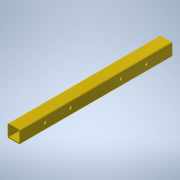
# Autodesk Inventor part: Lacznik prosty
Saved by Autodesk Inventor 2021 (Build 250183000, 183)
## iProperties
Created: 2024-04-08
Part Number: Lacznik prosty
Material: Steel
Document SubType Name: Modeling
Designer: Michal
Density: 7.85 g/cm^3
Appearance: Glossy - Gold
Author: Michal
Autodesk Inventor part; units mm, degrees
ref_plane "YZ Plane" through (0, 0, 0) normal (1, 0, 0) x (0, 1, 0)
ref_plane "XZ Plane" through (0, 0, 0) normal (0, 1, 0) x (-1, 0, 0)
ref_plane "XY Plane" through (0, 0, 0) normal (0, 0, 1) x (1, 0, 0)
sketch "Sketch1" plane through (0, 0, 0) normal (0, 1, 0) x (-1, 0, 0)
  line L0 (-9.5, 11.5) -> (9.5, 11.5) construction
  line L1 (11.5, 9.5) -> (11.5, -9.5) construction
  line L2 (9.5, -11.5) -> (-9.5, -11.5) construction
  line L3 (-11.5, -9.5) -> (-11.5, 9.5) construction
  line L4 (-11.5, 11.5) -> (11.5, -11.5) construction
  line L5 (11.5, 11.5) -> (-11.5, -11.5) construction
  arc A0 (11.5, 9.5) -> (9.5, 11.5) centre (9.5, 9.5) ccw construction
  arc A1 (9.5, -11.5) -> (11.5, -9.5) centre (9.5, -9.5) ccw construction
  arc A2 (-11.5, -9.5) -> (-9.5, -11.5) centre (-9.5, -9.5) ccw construction
  arc A3 (-9.5, 11.5) -> (-11.5, 9.5) centre (-9.5, 9.5) ccw construction
  line L6 (-9.5, -12.5) -> (9.5, -12.5)
  arc A4 (9.5, -12.5) -> (12.5, -9.5) centre (9.5, -9.5) ccw
  line L7 (12.5, -9.5) -> (12.5, 9.5)
  arc A5 (12.5, 9.5) -> (9.5, 12.5) centre (9.5, 9.5) ccw
  line L8 (9.5, 12.5) -> (-9.5, 12.5)
  arc A6 (-9.5, 12.5) -> (-12.5, 9.5) centre (-9.5, 9.5) ccw
  line L9 (-12.5, 9.5) -> (-12.5, -9.5)
  arc A7 (-12.5, -9.5) -> (-9.5, -12.5) centre (-9.5, -9.5) ccw
  line L10 (10.5, -9.5) -> (10.5, 9.5)
  arc A8 (10.5, 9.5) -> (9.5, 10.5) centre (9.5, 9.5) ccw
  line L11 (9.5, 10.5) -> (-9.5, 10.5)
  arc A9 (-9.5, 10.5) -> (-10.5, 9.5) centre (-9.5, 9.5) ccw
  line L12 (-10.5, 9.5) -> (-10.5, -9.5)
  arc A10 (-10.5, -9.5) -> (-9.5, -10.5) centre (-9.5, -9.5) ccw
  line L13 (-9.5, -10.5) -> (9.5, -10.5)
  arc A11 (9.5, -10.5) -> (10.5, -9.5) centre (9.5, -9.5) ccw
  point P0 (0, 0)
  point P1 (0, 0)
  point P2 (0, 0)
  dimension "d10" = 2
  dimension "depth" = 25
  dimension "width" = 25
  dimension "thickness" = 2
  constraints: 28 end point, 24 point on circle, 12 centre point, 8 point on line, 8 tangent, 6 parallel, 3 equal radius, 3 midpoint, 3 perpendicular, 1 coincident, 1 horizontal, 15 other
  measures "d10" radius of A0
  measures "depth" distance between parallel lines of L6 L8
  measures "width" distance between parallel lines of L9 L7
  measures "thickness" distance between parallel lines of L10 L7
extrude "Extrusion1" add sketch "Sketch1" along normal blind 300
sketch "Sketch2" plane through (12.5, 0, 9.5) normal (1, 0, 0) x (0, 0, -1)
  line L0 (9.5, -60) -> (9.5, 360) construction
  line L1 (0, 300) -> (19, 300) projected
  line L2 (0, 0) -> (19, 0) projected
  line L3 (-3, 0) -> (-3, 300) projected
  line L4 (-3, 150) -> (-40.443, 150) construction
  point P0 (9.5, 0)
  point P1 (9.5, 250)
  point P2 (9.5, 200)
  point P3 (9.5, 50)
  point P4 (9.5, 100)
  dimension "d17" = 50
  dimension "d28" = 50
  dimension "d29" = 100
  constraints: 4 point on line, 2 end point, 1 horizontal, 1 midpoint, 1 symmetric about line
  measures "d17" distance of point (9.5, 200) point (9.5, 250)
  measures "d28" distance of point (9.5, 100) point (9.5, 50)
  measures "d29" distance of point (9.5, 100) point (9.5, 200)
hole "Hole1" at (12.5, 250, 0) at (12.5, 200, 0) at (12.5, 100, 0) at (12.5, 50, 0) direction (-1, 0, 0) diameter 6.647 depth 20.2 tip angle 118 thread size "M8x1.25" class "6H" standard "ANSI Metric M Profile"
equation "\"d10\" = thickness"
body "Solid1"
